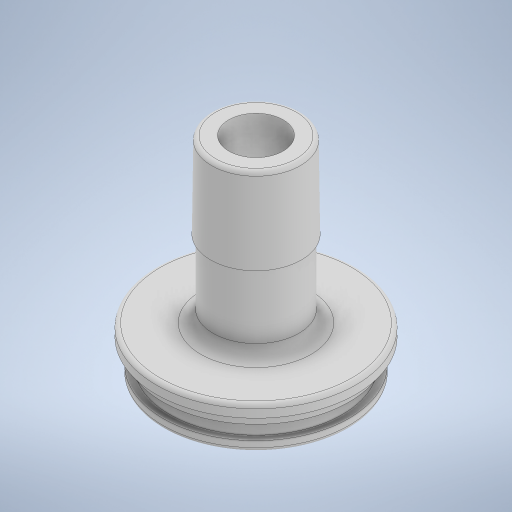
# Autodesk Inventor part: Rebreather-HoseAdapterInsert
Saved by Autodesk Inventor 2023 (Build 270158000, 158)
## iProperties
Created: 2022-11-09
Part Number: Rebreather-HoseAdapterInsert
Material: Generic
Document SubType Name: Modeling
Designer: incep
Density: 1 g/cm^3
Appearance: Default
Author: incep
## iProperties of the stored document Rebreather-HoseAdapterInsert_3DPrint.ipt
Created: 2022-11-09
Part Number: Rebreather-HoseAdapterInsert_3DPrint
Material: Generic
Document SubType Name: Modeling
Designer: incep
Density: 1 g/cm^3
Appearance: Default
Author: incep
Autodesk Inventor part; units mm, degrees
ref_plane "YZ Plane" through (0, 0, 0) normal (1, 0, 0) x (0, 1, 0)
ref_plane "XZ Plane" through (0, 0, 0) normal (0, 1, 0) x (-1, 0, 0)
ref_plane "XY Plane" through (0, 0, 0) normal (0, 0, 1) x (1, 0, 0)
sketch "Sketch1" plane through (0, 0, 0) normal (0, 0, 1) x (1, 0, 0)
  line L0 (-24.6, 0) -> (24.6, 0) construction
  line L1 (24.6, 0) -> (24.6, -3)
  line L2 (24.6, -3) -> (-24.6, -3) construction
  line L3 (-24.6, -3) -> (-24.6, 0)
  line L4 (-22.9, -3) -> (22.9, -3) construction
  line L5 (22.9, -3) -> (22.9, -11.5) construction
  line L6 (22.9, -11.5) -> (-22.9, -11.5) construction
  line L7 (-22.9, -11.5) -> (-22.9, -3)
  line L8 (22.9, -9) -> (21.25, -9)
  line L9 (21.25, -9) -> (21.25, -5.5)
  line L10 (21.25, -5.5) -> (22.9, -5.5)
  line L11 (22.9, -5.5) -> (22.9, -9) construction
  line L12 (-10.55, 40) -> (10.55, 40) construction
  line L13 (10.55, 40) -> (10.55, 0) construction
  line L14 (10.55, 0) -> (-10.55, 0) construction
  line L15 (-10.55, 0) -> (-10.55, 40) construction
  line L16 (-10.92, 40) -> (10.92, 40) construction
  line L17 (-11.19, 19) -> (11.19, 19) construction
  line L18 (-10.92, 40) -> (-11.19, 19)
  line L19 (10.92, 40) -> (11.19, 19)
  line L20 (-6.7, 40) -> (6.7, 40) construction
  line L21 (6.7, 40) -> (6.7, -3) construction
  line L22 (6.7, -3) -> (-6.7, -3) construction
  line L23 (-6.7, -3) -> (-6.7, 40) construction
  line L24 (-18.9, -3) -> (18.9, -3) construction
  line L25 (18.9, -3) -> (18.9, -11.5)
  line L26 (18.9, -11.5) -> (-18.9, -11.5) construction
  line L27 (-18.9, -11.5) -> (-18.9, -3)
  line L28 (-22.9, -11.5) -> (-18.9, -11.5)
  line L29 (18.9, -11.5) -> (22.9, -11.5)
  line L30 (-24.6, -3) -> (-22.9, -3)
  line L31 (-18.9, -3) -> (-6.7, -3)
  line L32 (6.7, -3) -> (18.9, -3)
  line L33 (22.9, -3) -> (24.6, -3)
  line L34 (22.9, -3) -> (22.9, -5.5)
  line L35 (22.9, -9) -> (22.9, -11.5)
  line L36 (10.55, 0) -> (24.6, 0)
  line L37 (-10.92, 40) -> (-6.7, 40)
  line L38 (6.7, 40) -> (10.92, 40)
  line L39 (10.55, 0) -> (10.55, 19)
  line L40 (10.55, 19) -> (11.19, 19)
  line L41 (-11.19, 19) -> (-10.55, 19)
  line L42 (-10.55, 19) -> (-10.55, 5.3907)
  line L43 (-6.7, 40) -> (-6.7, -3)
  line L44 (6.7, 40) -> (6.7, -3)
  line L45 (10.55, 0) -> (24.6, 0)
  line L46 (0, -21.8) -> (0, 50.3) projected
  point P0 (0, 0)
  point P1 (0, 0)
  point P2 (0, -3)
  point P3 (22.9, -7.25)
  point P4 (22.9, -7.25)
  point P5 (0, 0)
  point P6 (0, 40)
  point P7 (0, 19)
  point P8 (0, 40)
  point P9 (0, -11.5)
  point P10 (0, -3)
  point P11 (-22.9, -7.25)
  dimension "d0" = 49.2
  dimension "d1" = 3
  dimension "d2" = 45.8
  dimension "d3" = 8.5
  dimension "d4" = 3.5
  dimension "d5" = 1.65
  dimension "d6" = 40
  dimension "d7" = 21.1
  dimension "d8" = 21.84
  dimension "d9" = 22.38
  dimension "d10" = 21
  dimension "d11" = 13.4
  dimension "d12" = 4
  constraints: 92 end point, 17 collinear, 12 midpoint, 12 parallel, 10 horizontal, 9 perpendicular, 5 point on line, 5 vertical alignment, 3 coincident
  measures "d0" distance of L0.start L0.end
  measures "d1" distance of L0.end L1.end
  measures "d2" distance between parallel lines of L5 L7
  measures "d3" distance of L4.end L5.end
  measures "d4" distance of L8.end L9.end
  measures "d5" distance of L8.start L8.end
  measures "d6" distance of L12.end L13.end
  measures "d7" distance of L12.start L12.end
  measures "d8" distance of L16.start L16.end
  measures "d9" distance of L17.start L17.end
  measures "d10" distance between parallel lines of L17 L12
  measures "d11" distance between parallel lines of L21 L23
  measures "d12" distance from line of point (-22.9, -7.25) L27
revolve "Revolution1" add sketch "Sketch1" angle 360 about axis through (0, -10, 0) along (0, 1, 0)
fillet "Fillet1" radius 1 4 edges at (-10.92, 40, 0) (-24.6, 0, 0) (-22.9, -11.5, 0) (-18.9, -11.5, 0)
fillet "Fillet2" radius 3 3 edges at (-10.55, 0, 0) (-6.7, -3, 0) (-18.9, -3, 0)
body "Solid1"
